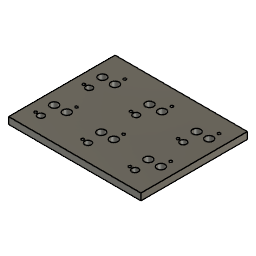
AC Box Outlet Connector Insert (Autodesk Fusion 360 design; units mm, degrees)
Autodesk Fusion 360 part; units mm, degrees
sketch "Sketch1" plane through (0, 0, 0) normal (0, 0, 1) x (1, 0, 0)
  circle A0 centre (120.0023, 74.4982) radius 17.7546
  circle A1 centre (32.3977, 74.4982) radius 17.5
  line L0 (137.5023, 101.6) -> (137.5023, 2.54)
  line L1 (14.8977, 56.9982) -> (14.8977, 91.9982)
  line L2 (102.5023, 56.9982) -> (102.5023, 91.9982)
  line L3 (93.7, 91.9982) -> (93.7, 56.9982)
  line L4 (49.8977, 91.9982) -> (49.8977, 56.9982)
  circle A2 centre (32.3977, 74.4982) radius 17.7546
  line L5 (14.6431, 74.4982) -> (14.6431, 2.54) construction
  circle A3 centre (76.2, 74.4982) radius 17.7546
  line L6 (137.5023, 56.9982) -> (137.5023, 91.9982) construction
  line L7 (14.8839, 2.54) -> (14.8839, 101.6)
  line L8 (76.2, 91.9982) -> (76.2, 56.9982) construction
  line L9 (49.8977, 56.9982) -> (14.8977, 56.9982)
  line L10 (50.1523, 74.4982) -> (50.1523, 2.54) construction
  line L11 (137.5023, 91.9982) -> (137.5023, 56.9982)
  line L12 (137.5023, 2.54) -> (14.8839, 2.54)
  line L13 (14.8839, 101.6) -> (137.5023, 101.6)
  line L14 (93.7, 29.6418) -> (93.7, 47.1418) construction
  line L15 (137.5023, 56.9982) -> (102.5023, 56.9982)
  line L16 (93.7, 12.1418) -> (93.7, 47.1418) construction
  circle A4 centre (120.0023, 29.6418) radius 17.5
  line L17 (137.5023, 29.6418) -> (137.5023, 47.1418) construction
  line L18 (137.5023, 47.1418) -> (137.5023, 12.1418)
  line L19 (58.4454, 74.4982) -> (58.4454, 2.54) construction
  line L20 (120.0023, 47.1418) -> (120.0023, 29.6418) construction
  line L21 (76.2, 47.1418) -> (76.2, 12.1418) construction
  line L22 (120.0023, 74.4982) -> (137.5023, 74.4982) construction
  line L23 (93.7, 47.1418) -> (76.2, 47.1418) construction
  line L24 (120.0023, 74.4982) -> (146.05, 74.4982) construction
  circle A5 centre (120.0023, 29.6418) radius 17.7546
  line L25 (137.5023, 47.1418) -> (120.0023, 47.1418) construction
  line L26 (93.7, 47.1418) -> (93.7, 12.1418)
  circle A6 centre (72.771, 18.3103) radius 3
  line L27 (93.9546, 74.4982) -> (93.9546, 2.54) construction
  circle A7 centre (114.1712, 33.0392) radius 3.7
  circle A8 centre (81.9707, 33.1238) radius 3.7
  line L28 (120.0023, 47.1418) -> (120.0023, 12.1418) construction
  line L29 (58.7, 29.6418) -> (93.7, 29.6418) construction
  circle A9 centre (125.773, 33.1238) radius 3.7
  line L30 (102.5023, 29.6418) -> (137.5023, 29.6418) construction
  line L31 (76.2, 47.1418) -> (76.2, 29.6418) construction
  circle A10 centre (116.5733, 18.3103) radius 3
  circle A11 centre (111.2632, 63.5652) radius 1.25
  circle A12 centre (76.2, 29.6418) radius 17.7546
  circle A13 centre (67.4609, 63.5652) radius 1.25
  line L32 (102.2477, 74.4982) -> (102.2477, 2.54) construction
  line L33 (76.2, 29.6418) -> (93.7, 29.6418) construction
  line L34 (102.5023, 74.4982) -> (137.5023, 74.4982) construction
  line L35 (120.0023, 29.6418) -> (137.5023, 29.6418) construction
  circle A14 centre (70.3689, 33.0392) radius 3.7
  circle A15 centre (67.4609, 18.7088) radius 1.25
  circle A16 centre (38.1684, 33.1238) radius 3.7
  circle A17 centre (70.3689, 77.8956) radius 3.7
  line L36 (93.7, 91.9982) -> (76.2, 91.9982) construction
  circle A18 centre (28.9687, 63.1667) radius 3
  line L37 (76.2, 91.9982) -> (76.2, 74.4982) construction
  circle A19 centre (120.0023, 74.4982) radius 17.5
  circle A20 centre (76.2, 74.4982) radius 17.5
  circle A21 centre (81.9707, 77.9802) radius 3.7
  line L38 (32.3977, 74.4982) -> (49.8977, 74.4982) construction
  line L39 (58.7, 12.1418) -> (58.7, 47.1418)
  circle A22 centre (23.6586, 63.5652) radius 1.25
  line L40 (49.8977, 12.1418) -> (14.8977, 12.1418)
  line L41 (120.0023, 101.6) -> (120.0023, 74.4982) construction
  line L42 (14.8977, 91.9982) -> (49.8977, 91.9982)
  line L43 (14.8977, 47.1418) -> (49.8977, 47.1418)
  circle A23 centre (28.9687, 18.3103) radius 3
  line L44 (137.5023, 91.9982) -> (120.0023, 91.9982) construction
  circle A24 centre (38.5383, 41.8839) radius 1.25
  line L45 (32.3977, 47.1418) -> (32.3977, 12.1418) construction
  circle A25 centre (114.1712, 77.8956) radius 3.7
  circle A26 centre (26.5666, 33.0392) radius 3.7
  circle A27 centre (126.1429, 86.7403) radius 1.25
  line L46 (102.5023, 91.9982) -> (137.5023, 91.9982)
  line L47 (32.3977, 91.9982) -> (32.3977, 74.4982) construction
  line L48 (49.8977, 91.9982) -> (32.3977, 91.9982) construction
  line L49 (58.7, 91.9982) -> (93.7, 91.9982)
  line L50 (14.6431, 101.6) -> (14.6431, 92.2528) construction
  line L51 (14.8977, 91.9982) -> (14.8839, 101.6) construction
  line L52 (76.2, 74.4982) -> (93.7, 74.4982) construction
  line L53 (137.7569, 74.4982) -> (137.7569, 2.54) construction
  line L54 (102.5023, 47.1418) -> (137.5023, 47.1418)
  line L55 (58.7, 74.4982) -> (93.7, 74.4982) construction
  line L56 (137.5023, 12.1418) -> (137.5023, 47.1418) construction
  circle A28 centre (126.1429, 41.8839) radius 1.25
  circle A29 centre (111.2632, 18.7088) radius 1.25
  circle A30 centre (82.3406, 41.8839) radius 1.25
  circle A31 centre (116.5733, 63.1667) radius 3
  circle A32 centre (72.771, 63.1667) radius 3
  line L57 (58.7, 47.1418) -> (93.7, 47.1418)
  line L58 (102.5023, 12.1418) -> (102.5023, 47.1418)
  circle A33 centre (76.2, 29.6418) radius 17.5
  line L59 (93.7, 12.1418) -> (58.7, 12.1418)
  line L60 (137.5023, 12.1418) -> (102.5023, 12.1418)
  line L61 (93.7, 56.9982) -> (58.7, 56.9982)
  line L62 (120.0023, 91.9982) -> (120.0023, 74.4982) construction
  line L63 (137.5023, 74.4982) -> (137.5023, 91.9982) construction
  line L64 (32.3977, 91.9982) -> (32.3977, 56.9982) construction
  line L65 (93.7, 74.4982) -> (93.7, 91.9982) construction
  line L66 (120.0023, 91.9982) -> (120.0023, 56.9982) construction
  line L67 (49.8977, 56.9982) -> (49.8977, 91.9982) construction
  circle A34 centre (32.3977, 29.6418) radius 17.7546
  circle A35 centre (38.1684, 77.9802) radius 3.7
  circle A36 centre (32.3977, 29.6418) radius 17.5
  line L68 (14.8977, 12.1418) -> (14.8977, 47.1418)
  line L69 (32.3977, 101.6) -> (32.3977, 74.4982) construction
  line L70 (58.7, 56.9982) -> (58.7, 91.9982)
  line L71 (14.8977, 29.6418) -> (49.8977, 29.6418) construction
  line L72 (32.3977, 2.54) -> (32.3977, 29.6418) construction
  line L73 (49.8977, 74.4982) -> (49.8977, 91.9982) construction
  line L74 (49.8977, 47.1418) -> (32.3977, 47.1418) construction
  line L75 (14.8977, 74.4982) -> (49.8977, 74.4982) construction
  line L76 (32.3977, 47.1418) -> (32.3977, 29.6418) construction
  circle A37 centre (23.6586, 18.7088) radius 1.25
  line L77 (49.8977, 47.1418) -> (49.8977, 12.1418)
  line L78 (49.8977, 12.1418) -> (49.8977, 47.1418) construction
  line L79 (49.8977, 29.6418) -> (49.8977, 47.1418) construction
  circle A38 centre (26.5666, 77.8956) radius 3.7
  circle A39 centre (38.5383, 86.7403) radius 1.25
  line L80 (32.3977, 29.6418) -> (49.8977, 29.6418) construction
  circle A40 centre (82.3406, 86.7403) radius 1.25
  line L81 (32.3977, 74.4982) -> (120.0023, 74.4982) construction
  line L82 (93.7, 56.9982) -> (93.7, 91.9982) construction
  circle A41 centre (125.773, 77.9802) radius 3.7
  line L83 (137.7569, 74.4982) -> (137.7569, 101.6) construction
  line L84 (14.6431, 2.54) -> (137.7569, 2.54)
  line L85 (137.7569, 2.54) -> (137.7569, 101.6)
  line L86 (137.7569, 101.6) -> (14.6431, 101.6)
  line L87 (14.6431, 101.6) -> (14.6431, 2.54)
  point P0 (88.9, 0)
  point P1 (32.3977, 74.4982)
  point P2 (38.5383, 86.7403)
  point P3 (32.3977, 29.6418)
  point P4 (38.5383, 41.8839)
  point P5 (82.3406, 86.7403)
  point P6 (76.2, 74.4982)
  point P7 (76.2, 29.6418)
  point P8 (82.3406, 41.8839)
  point P9 (120.0023, 29.6418)
  point P10 (126.1429, 41.8839)
  point P11 (120.0023, 74.4982)
  point P12 (126.1429, 86.7403)
  dimension "d117" = -87.6046
  dimension "d118" = -44.8564
  dimension "d123" = 35.5092
  dimension "d126" = 27.1018
  dimension "d127" = 87.6046
  dimension "d128" = 44.8564
  dimension "d129" = 2.5
  dimension "d130" = 35
  dimension "d131" = 2.5
  dimension "d132" = 7.4
  dimension "d133" = 7.4
  dimension "d134" = 6
  dimension "d135" = 12.2421
  dimension "d136" = 6.1406
  dimension "d137" = 5.7707
  dimension "d139" = 5.8311
  dimension "d140" = 11.3315
  dimension "d141" = 3.482
  dimension "d142" = 8.7391
  dimension "d143" = 10.933
  dimension "d144" = 3.429
  dimension "d145" = 35
  dimension "d146" = 2.5
  dimension "d147" = 35
  dimension "d148" = 2.5
  dimension "d149" = 7.4
  dimension "d150" = 7.4
  dimension "d151" = 6
  dimension "d152" = 12.2421
  dimension "d153" = 6.1406
  dimension "d154" = 5.7707
  dimension "d155" = 3.3974
  dimension "d156" = 5.8311
  dimension "d157" = 11.3315
  dimension "d158" = 3.482
  dimension "d159" = 8.7391
  dimension "d160" = 10.933
  dimension "d161" = 3.429
  dimension "d162" = 35
  dimension "d163" = 2.5
  dimension "d164" = 35
  dimension "d165" = 2.5
  dimension "d166" = 7.4
  dimension "d167" = 7.4
  dimension "d168" = 6
  dimension "d169" = 12.2421
  dimension "d170" = 6.1406
  dimension "d171" = 5.7707
  dimension "d173" = 5.8311
  dimension "d174" = 11.3315
  dimension "d175" = 3.482
  dimension "d176" = 8.7391
  dimension "d177" = 10.933
  dimension "d178" = 3.429
  dimension "d179" = 35
  dimension "d180" = 2.5
  dimension "d181" = 35
  dimension "d182" = 2.5
  dimension "d183" = 7.4
  dimension "d184" = 7.4
  dimension "d185" = 6
  dimension "d186" = 12.2421
  dimension "d187" = 6.1406
  dimension "d188" = 5.7707
  dimension "d189" = 3.3974
  dimension "d190" = 5.8311
  dimension "d191" = 11.3315
  dimension "d192" = 3.482
  dimension "d193" = 8.7391
  dimension "d194" = 10.933
  dimension "d195" = 3.429
  dimension "d196" = 35
  dimension "d197" = 2.5
  dimension "d198" = 35
  dimension "d199" = 2.5
  dimension "d200" = 7.4
  dimension "d201" = 7.4
  dimension "d202" = 6
  dimension "d203" = 12.2421
  dimension "d204" = 6.1406
  dimension "d205" = 5.7707
  dimension "d206" = 3.3974
  dimension "d207" = 5.8311
  dimension "d208" = 11.3315
  dimension "d209" = 3.482
  dimension "d210" = 8.7391
  dimension "d211" = 10.933
  dimension "d212" = 3.429
  dimension "d213" = 35
  dimension "d214" = 2.5
  dimension "d215" = 35
  dimension "d216" = 2.5
  dimension "d217" = 7.4
  dimension "d218" = 7.4
  dimension "d219" = 6
  dimension "d220" = 12.2421
  dimension "d221" = 6.1406
  dimension "d222" = 5.7707
  dimension "d223" = 3.3974
  dimension "d224" = 5.8311
  dimension "d225" = 11.3315
  dimension "d226" = 3.482
  dimension "d227" = 8.7391
  dimension "d228" = 10.933
  dimension "d229" = 3.429
  constraint vertical L50
  constraint vertical L41
  constraint horizontal L24
  constraint coincident P11 A0.centre
  constraint vertical L69
  constraint coincident L10.start A2
  constraint coincident L10.start L81
  constraint tangent A2 L10
  constraint coincident L5.start A2
  constraint tangent A2 L5
  constraint coincident L19.start A3
  constraint coincident L19.start L81
  constraint tangent A3 L19
  constraint coincident L27.start L81
  constraint coincident L27.start A3
  constraint tangent A3 L27
  constraint coincident L32.start A0
  constraint coincident L32.start L81
  constraint tangent A0 L32
  constraint coincident L53.start A0
  constraint coincident L53.start L24
  constraint tangent A0 L53
  constraint coincident P2 A39.centre
  constraint midpoint P1 L75
  constraint coincident P1 A1.centre
  constraint coincident L38.end A1
  constraint horizontal L75
  constraint perpendicular L38 L73
  constraint parallel L38 L48
  constraint parallel L47 L73
  constraint parallel L38 L75
  constraint midpoint L38.end L67
  constraint perpendicular L4 L9
  constraint parallel L1 L4
  constraint parallel L9 L42
  constraint midpoint L64.end L9
  constraint perpendicular L9 L64
  constraint coincident P5 A40.centre
  constraint midpoint P6 L55
  constraint coincident P6 A3.centre
  constraint coincident L52.end A20
  constraint horizontal L55
  constraint perpendicular L52 L65
  constraint parallel L36 L52
  constraint parallel L37 L65
  constraint parallel L52 L55
  constraint midpoint L52.end L82
  constraint perpendicular L3 L61
  constraint parallel L3 L70
  constraint parallel L49 L61
  constraint midpoint L8.end L61
  constraint perpendicular L8 L61
  constraint coincident P4 A24.centre
  constraint midpoint P3 L71
  constraint coincident P3 A34.centre
  constraint coincident L71.end A36
  constraint horizontal L71
  constraint perpendicular L79 L80
  constraint parallel L74 L80
  constraint parallel L76 L79
  constraint parallel L71 L80
  constraint midpoint L71.end L78
  constraint perpendicular L40 L77
  constraint parallel L68 L77
  constraint parallel L40 L43
  constraint midpoint L45.end L40
  constraint perpendicular L40 L45
  constraint coincident P8 A30.centre
  constraint midpoint P7 L29
  constraint coincident P7 L31.end
  constraint coincident L14.start A33
  constraint horizontal L29
  constraint perpendicular L14 L33
  constraint parallel L23 L33
  constraint parallel L14 L31
  constraint parallel L29 L33
  constraint midpoint L14.start L16
  constraint perpendicular L26 L59
  constraint parallel L26 L39
  constraint parallel L57 L59
  constraint midpoint L21.end L59
  constraint perpendicular L21 L59
  constraint coincident P10 A28.centre
  constraint midpoint P9 L30
  constraint coincident P9 A4.centre
  constraint coincident L17.start A4
  constraint horizontal L30
  constraint perpendicular L17 L35
  constraint parallel L25 L35
  constraint parallel L17 L20
  constraint parallel L30 L35
  constraint midpoint L17.start L56
  constraint perpendicular L18 L60
  constraint parallel L18 L58
  constraint parallel L54 L60
  constraint midpoint L28.end L60
  constraint perpendicular L28 L60
  constraint coincident P12 A27.centre
  constraint midpoint P11 L34
  constraint coincident L22.end A19
  constraint horizontal L34
  constraint perpendicular L22 L63
  constraint parallel L22 L44
  constraint parallel L62 L63
  constraint parallel L22 L34
  constraint midpoint L22.end L6
  constraint perpendicular L11 L15
  constraint parallel L2 L11
  constraint parallel L15 L46
  constraint midpoint L66.end L15
  constraint perpendicular L15 L66
  constraint horizontal L13
  constraint vertical L0
  constraint horizontal L12
  constraint vertical L7
  constraint tangent A0 L83
  constraint horizontal L84
  constraint vertical L85
  constraint horizontal L86
  constraint vertical L87
  measures "d123" diameter of A0
  measures "d126" distance of P3 L72.start
  measures "d127" distance of P11 P1
  measures "d128" distance of P1 P3
  measures "d129" diameter of A39
  measures "d130" diameter of A1
  measures "d131" diameter of A22
  measures "d132" diameter of A35
  measures "d133" diameter of A38
  measures "d134" diameter of A18
  measures "d135" vertical distance of P1 P2
  measures "d136" horizontal distance of P1 P2
  measures "d137" horizontal distance of P1 A35.centre
  measures "d139" horizontal distance of A38.centre P1
  measures "d140" vertical distance of P1 A18.centre
  measures "d141" vertical distance of P1 A35.centre
  measures "d142" horizontal distance of A22.centre P1
  measures "d143" vertical distance of A22.centre P1
  measures "d144" horizontal distance of P1 A18.centre
  measures "d145" distance of L4.start L4.end
  measures "d146" diameter of A40
  measures "d147" diameter of A20
  measures "d148" diameter of A13
  measures "d149" diameter of A21
  measures "d150" diameter of A17
  measures "d151" diameter of A32
  measures "d152" vertical distance of P6 P5
  measures "d153" horizontal distance of P6 P5
  measures "d154" horizontal distance of A21.centre P6
  measures "d155" vertical distance of A17.centre P6
  measures "d156" horizontal distance of A17.centre P6
  measures "d157" vertical distance of A32.centre P6
  measures "d158" vertical distance of A21.centre P6
  measures "d159" horizontal distance of A13.centre P6
  measures "d160" vertical distance of A13.centre P6
  measures "d161" horizontal distance of A32.centre P6
  measures "d162" distance of L3.start L3.end
  measures "d163" diameter of A24
  measures "d164" diameter of A36
  measures "d165" diameter of A37
  measures "d166" diameter of A16
  measures "d167" diameter of A26
  measures "d168" diameter of A23
  measures "d169" vertical distance of P3 P4
  measures "d170" horizontal distance of P3 P4
  measures "d171" horizontal distance of P3 A16.centre
  measures "d173" horizontal distance of A26.centre P3
  measures "d174" vertical distance of A23.centre P3
  measures "d175" vertical distance of P3 A16.centre
  measures "d176" horizontal distance of A37.centre P3
  measures "d177" vertical distance of A37.centre P3
  measures "d178" horizontal distance of A23.centre P3
  measures "d179" distance of L43.end L40.start
  measures "d180" diameter of A30
  measures "d181" diameter of A33
  measures "d182" diameter of A15
  measures "d183" diameter of A8
  measures "d184" diameter of A14
  measures "d185" diameter of A6
  measures "d186" vertical distance of P7 P8
  measures "d187" horizontal distance of P7 P8
  measures "d188" horizontal distance of P7 A8.centre
  measures "d189" vertical distance of P7 A14.centre
  measures "d190" horizontal distance of P7 A14.centre
  measures "d191" vertical distance of A6.centre P7
  measures "d192" vertical distance of P7 A8.centre
  measures "d193" horizontal distance of P7 A15.centre
  measures "d194" vertical distance of P7 A15.centre
  measures "d195" horizontal distance of A6.centre P7
  measures "d196" distance of L16.start L14.end
  measures "d197" diameter of A28
  measures "d198" diameter of A4
  measures "d199" diameter of A29
  measures "d200" diameter of A9
  measures "d201" diameter of A7
  measures "d202" diameter of A10
  measures "d203" vertical distance of P9 P10
  measures "d204" horizontal distance of P9 P10
  measures "d205" horizontal distance of P9 A9.centre
  measures "d206" vertical distance of A7.centre P9
  measures "d207" horizontal distance of A7.centre P9
  measures "d208" vertical distance of A10.centre P9
  measures "d209" vertical distance of P9 A9.centre
  measures "d210" horizontal distance of A29.centre P9
  measures "d211" vertical distance of A29.centre P9
  measures "d212" horizontal distance of A10.centre P9
  measures "d213" distance of L17.end L18.end
  measures "d214" diameter of A27
  measures "d215" diameter of A19
  measures "d216" diameter of A11
  measures "d217" diameter of A41
  measures "d218" diameter of A25
  measures "d219" diameter of A31
  measures "d220" vertical distance of P11 P12
  measures "d221" horizontal distance of P11 P12
  measures "d222" horizontal distance of P11 A41.centre
  measures "d223" vertical distance of P11 A25.centre
  measures "d224" horizontal distance of P11 A25.centre
  measures "d225" vertical distance of P11 A31.centre
  measures "d226" vertical distance of P11 A41.centre
  measures "d227" horizontal distance of P11 A11.centre
  measures "d228" vertical distance of P11 A11.centre
  measures "d229" horizontal distance of P11 A31.centre
extrude "Extrude1" add sketch "Sketch1" along normal blind 6.35 contours A0 L0 L11 | A0 L0 L11 L18 A5 L85 | A0 L0 L11 L85 L86 | A0 L0 L11 A19 L46 | A0 L0 L11 L46 | A0 L0 L11 L15 | A0 L0 L11 L15 A19 | L0 L18 A5 | L0 L18 A5 L84 L85 | A0 L46 | A0 L0 L1 L2 L4 A2 L7 L9 L12 L13 L15 A5 L40 L42 L43 L46 L54 L58 L60 A34 L68 L77 L84 L86 | A19 | A0 L15 | L0 L18 A5 L54 | L0 A4 L18 A5 L54 | L0 A4 L18 A5 L60 | L0 L18 A5 L60 | A0 L2 A19 L46 | A0 L2 L46 | A0 L2 L15 A19 | A0 L2 L15 | A4 | A5 L54 | A5 L60 | A2 L7 L86 L87 | A0 L2 | A4 A5 L54 L58 | A4 A5 L58 L60 | A5 L54 L58 | A5 L58 L60 | L7 A34 L84 L87 | A2 L7 | L1 A2 L7 | A5 L58 | L7 A34 | L7 A34 L68 | A1 L1 A2 L42 | L1 A2 L42 | A2 L7 A34 L87 | L40 A34 A36 L68 | L40 A34 L68 | A1 | A1 L1 A2 L9 | A2 L42 | L1 A2 L9 | L43 A34 L68 | L43 A34 A36 L68 | L40 A34 | A36 | A1 L4 A2 L42 | A1 L4 A2 L9 | A2 L9 | L4 A2 L42 | L43 A34 | L40 A34 A36 L77 | L40 A34 L77 | L43 A34 A36 L77 | L4 A2 | L4 A2 L9 | L43 A34 L77 | A34 L77 | L3 A3 L49 | L3 A3 | L3 A3 A20 L49 | A3 L49 | A20 | L3 A3 A20 L61 | A3 A20 L49 L70 | A3 L49 L70 | L3 A3 L61 | A3 A20 L61 L70 | A3 L61 | A3 L70 | A3 L61 L70 | L26 A12 L57 | L26 A12 | L26 A12 L57 A33 | A12 L57 | A33 | L26 A12 A33 L59 | A12 L39 L57 A33 | A12 L39 L57 | L26 A12 L59 | A12 L39 A33 L59 | A12 L59 | A12 L39 | A12 L39 L59
